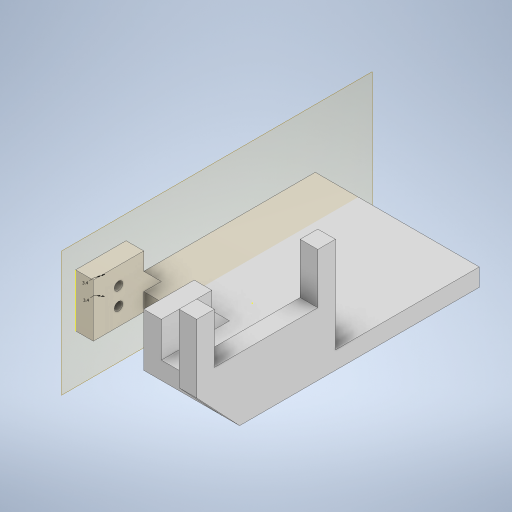
# Autodesk Inventor part: graber thingie
Saved by Autodesk Inventor 2024 (Build 280153020, 153B)
## iProperties
Created: 2023-12-18
Part Number: graber thingie
Material: Generic
Document SubType Name: Modeling
Designer: 5802269
Density: 1 g/cm^3
Appearance: Default
Author: 5802269
Autodesk Inventor part; units mm, degrees
ref_plane "YZ Plane" through (0, 0, 0) normal (1, 0, 0) x (0, 1, 0)
ref_plane "XZ Plane" through (0, 0, 0) normal (0, 1, 0) x (-1, 0, 0)
ref_plane "XY Plane" through (0, 0, 0) normal (0, 0, 1) x (1, 0, 0)
sketch "Sketch1" plane through (0, 0, 0) normal (0, 1, 0) x (-1, 0, 0)
  line L0 (32.5, 37.5) -> (-32.5, 37.5)
  line L1 (-32.5, 37.5) -> (-32.5, -37.5)
  line L2 (-32.5, -37.5) -> (32.5, -37.5)
  line L3 (32.5, -37.5) -> (32.5, 37.5)
  line L4 (32.5, 37.5) -> (-32.5, -37.5) construction
  line L5 (-32.5, 37.5) -> (32.5, -37.5) construction
  point P0 (0, 0)
  dimension "d0" = 65
  dimension "d1" = 75
  constraints: 12 end point, 2 midpoint, 2 parallel, 1 horizontal, 1 perpendicular
  measures "d0" distance of L2.end L1.end
  measures "d1" distance of L1.end L0.end
extrude "Extrusion1" add sketch "Sketch1" along normal blind 7
sketch "Sketch6" plane through (0, 7, 0) normal (0, 1, 0) x (1, 0, 0)
  line L0 (-32.5, 37.5) -> (-32.5, -37.5) projected
  line L1 (-32.5, -37.5) -> (-25.5, -37.5)
  line L2 (-32.5, -37.5) -> (32.5, -37.5) projected
  line L3 (-25.5, -37.5) -> (-25.5, -17.5)
  line L4 (-25.5, -17.5) -> (-5.5, -17.5)
  line L5 (-5.5, -17.5) -> (-5.5, -37.5)
  line L6 (-25.5, -17.5) -> (-32.5, -17.5)
  point P0 (0, 0)
  dimension "d13" = 7
  dimension "d14" = 20
  dimension "d15" = 20
  dimension "d16" = 20
  dimension "d17" = 90
  constraints: 10 end point, 4 perpendicular, 2 point on line
  measures "d13" distance of L0.end L1.end
  measures "d14" distance of L1.end L3.end
  measures "d15" distance of L3.end L4.end
  measures "d16" distance of L4.end L5.end
  measures "d17" angle of L4 L5
extrude "Extrusion4" cut sketch "Sketch6" against normal blind 14 contours L4 L5 L2 L3
sketch "Sketch7" plane through (0, 7, 0) normal (0, 1, 0) x (1, 0, 0)
  line L0 (-25.5, -37.5) -> (-25.5, -17.5) projected
  line L1 (-32.5, -37.5) -> (-25.5, -37.5)
  line L2 (-25.5, -37.5) -> (-25.5, -17.5)
  line L3 (-25.5, -17.5) -> (-32.5, -17.5)
  line L4 (-32.5, -17.5) -> (-32.5, -37.5)
  point P0 (0, 0)
  constraints: 8 end point, 2 parallel, 1 horizontal, 1 perpendicular
extrude "Extrusion5" add sketch "Sketch7" along normal blind 14
sketch "Sketch8" plane through (0, 7, 0) normal (0, 1, 0) x (1, 0, 0)
  line L0 (-5.5, -37.5) -> (32.5, -37.5) projected
  line L1 (32.5, -37.5) -> (25.5, -37.5)
  line L2 (25.5, -37.5) -> (25.5, 0.5)
  line L3 (25.5, 0.5) -> (32.5, 0.5)
  line L4 (32.5, 0.5) -> (32.5, -37.5)
  point P0 (0, 0)
  dimension "d22" = 7
  dimension "d23" = 38
  constraints: 8 end point, 2 parallel, 1 horizontal, 1 perpendicular
  measures "d22" distance of L2.end L3.end
  measures "d23" distance of L1.end L2.end
extrude "Extrusion6" add sketch "Sketch8" along normal blind 18
sketch "Sketch9" plane through (0, 25, 0) normal (0, 1, 0) x (1, 0, 0)
  line L0 (32.5, 0.5) -> (25.5, 0.5) projected
  line L1 (25.5, 0.5) -> (25.5, -37.5) projected
  line L2 (32.5, 0.5) -> (25.5, 0.5)
  line L3 (25.5, 0.5) -> (25.5, -6.5)
  line L4 (25.5, -6.5) -> (32.5, -6.5)
  line L5 (32.5, -6.5) -> (32.5, 0.5)
  point P0 (0, 0)
  dimension "d26" = 7
  constraints: 8 end point, 2 parallel, 1 horizontal, 1 perpendicular, 1 point on line
  measures "d26" distance of L3.end L2.end
extrude "Extrusion7" add sketch "Sketch9" along normal blind 20
sketch "Sketch10" plane through (0, 25, 0) normal (0, 1, 0) x (1, 0, 0)
  line L0 (32.5, -6.5) -> (32.5, 0.5) projected
  line L1 (32.5, 0.5) -> (32.5, -54.5)
  line L2 (32.5, -54.5) -> (25.5, -54.5)
  line L3 (25.5, -54.5) -> (25.5, -47.5)
  line L4 (25.5, -47.5) -> (32.5, -47.5)
  line L5 (32.5, -47.5) -> (32.5, -54.5)
  point P0 (0, 0)
  dimension "d29" = 55
  dimension "d30" = 7
  dimension "d31" = 7
  constraints: 10 end point, 2 parallel, 1 collinear, 1 horizontal, 1 perpendicular
  measures "d29" distance of L0.end L1.end
  measures "d30" distance of L3.end L4.end
  measures "d31" distance of L2.end L3.end
extrude "Extrusion8" add sketch "Sketch10" along normal blind 20
sketch "Sketch11" plane through (32.5, 0, 37.5) normal (1, 0, 0) x (0, 0, -1)
  line L0 (-17, 25) -> (-10, 25) projected
  line L1 (0, 7) -> (0, 25) construction
  line L2 (0, 7) -> (0, 25)
  line L3 (0, 25) -> (-17, 25)
  line L4 (-17, 25) -> (-17, 45) projected
  line L5 (0, 7) -> (0, 0)
  line L6 (-17, 25) -> (-17, 18)
  line L7 (-17, 18) -> (0, 0)
  point P0 (37.5, 0)
  dimension "d37" = 7
  constraints: 10 end point, 2 perpendicular, 1 collinear, 1 vertical
  measures "d37" distance of L0.start L6.end
extrude "Extrusion9" add sketch "Sketch11" against normal up to surface (7 mm away)
sketch "Sketch13" plane through (32.5, 0, -37.5) normal (0, 0, -1) x (-1, 0, 0)
  line L0 (65, 7) -> (58, 7) projected
  line L1 (0, 0) -> (65, 0)
  line L2 (65, 0) -> (65, 7)
  line L3 (65, 7) -> (0, 7)
  line L4 (0, 7) -> (0, 0)
  point P0 (32.5, 0)
  constraints: 8 end point, 2 parallel, 1 horizontal, 1 perpendicular
extrude "Extrusion10" add sketch "Sketch13" along normal blind 20
sketch "Sketch14" plane through (0, 7, 0) normal (0, 1, 0) x (1, 0, 0)
  point P0 (0, 0)
sketch "Sketch15" plane through (-25.5, 0, 37.5) normal (1, 0, 0) x (0, 0, -1)
  point P0 (37.5, 0)
sketch "Sketch16" plane through (-32.5, 0, 37.5) normal (-1, 0, 0) x (0, 0, 1)
  point P0 (-37.5, 0)
ref_plane "Work Plane1" through (-15.5, 0, 37.5) normal (1, 0, 0) x (0, 0, -1)
mirror "Mirror1" about plane through (-15.5, 0, 37.5) normal (1, 0, 0) of "Extrusion5"
sketch "Sketch18" plane through (-32.5, 0, 37.5) normal (-1, 0, 0) x (0, 0, 1)
  line L0 (-20, 7) -> (-20, 0) projected
  line L1 (-20, 7) -> (-20, 14)
  line L2 (-20, 7) -> (-20, 21) projected
  line L3 (-20, 7) -> (-13, 7) construction
  line L4 (-20, 14) -> (-27, 7)
  line L5 (-20, 7) -> (-95, 7) projected
  point P0 (-37.5, 0)
  dimension "d43" = 7
  dimension "d44" = 90
  dimension "d45" = 45
  constraints: 6 end point, 1 collinear, 1 horizontal, 1 perpendicular, 1 point on line
  measures "d43" distance of L0.start L1.end
  measures "d44" angle of L3 L1
  measures "d45" angle of L4 L1
extrude "Extrusion12" add sketch "Sketch18" against normal up to surface (7 mm away)
mirror "Mirror2" about plane through (-15.5, 0, 37.5) normal (1, 0, 0) of "Extrusion12"
sketch "Sketch19" plane through (-32.5, 0, 37.5) normal (-1, 0, 0) x (0, 0, 1)
  line L0 (0, 0) -> (0, 21) projected
  line L1 (-20, 14) -> (-20, 21) projected
  circle A0 centre (-10, 14) radius 1.7 construction
  circle A1 centre (-10, 7) radius 1.7 construction
  point P0 (-37.5, 0)
  dimension "d52" = 3.4
  dimension "d53" = 3.4
  constraints: 2 centre point
  measures "d52" diameter of A0
  measures "d53" diameter of A1
sketch "Sketch20" plane through (-32.5, 0, 37.5) normal (-1, 0, 0) x (0, 0, 1)
  line L0 (0, 7) -> (-38, 7) projected
  circle A0 centre (-9.9905, 7) radius 1.7
  circle A1 centre (-9.9905, 13.9998) radius 1.7
  point P0 (-37.5, 0)
  dimension "d54" = 3.4
  dimension "d55" = 3.4
  constraints: 2 centre point, 1 point on line
  measures "d54" diameter of A0
  measures "d55" diameter of A1
extrude "Extrusion13" cut sketch "Sketch20" against normal up to surface (34 mm away)
body "Solid1"
